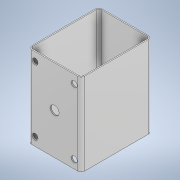
# Autodesk Inventor part: SP21V1 Tubo 40x80x100mm
Saved by Autodesk Inventor 2021.2 (Build 252289000, 289)
## iProperties
Created: 2026-06-02
Part Number: SP21V1 Tubo 40x80x100mm
Material: Aluminum
Document SubType Name: Modeling
Designer: nelso
Density: 2.7 g/cm^3
Appearance: Satin
Author: nelso
Autodesk Inventor part; units mm, degrees
ref_plane "YZ Plane" through (0, 0, 0) normal (1, 0, 0) x (0, 1, 0)
ref_plane "XZ Plane" through (0, 0, 0) normal (0, 1, 0) x (-1, 0, 0)
ref_plane "XY Plane" through (0, 0, 0) normal (0, 0, 1) x (1, 0, 0)
sketch "Sketch1" plane through (0, 0, 0) normal (0, 1, 0) x (-1, 0, 0)
  line L0 (-30, 40) -> (30, 40)
  line L1 (30, 40) -> (30, -40)
  line L2 (30, -40) -> (-30, -40)
  line L3 (-30, -40) -> (-30, 40)
  line L4 (-30, 40) -> (30, -40) construction
  line L5 (30, 40) -> (-30, -40) construction
  line L6 (-28.75, 38.75) -> (28.75, 38.75)
  line L7 (28.75, 38.75) -> (28.75, -38.75)
  line L8 (28.75, -38.75) -> (-28.75, -38.75)
  line L9 (-28.75, -38.75) -> (-28.75, 38.75)
  line L10 (-28.75, 38.75) -> (28.75, -38.75) construction
  line L11 (28.75, 38.75) -> (-28.75, -38.75) construction
  point P0 (0, 0)
  dimension "d0" = 60
  dimension "d1" = 80
  dimension "d2" = 57.5
  dimension "d3" = 77.5
  constraints: 24 end point, 4 midpoint, 4 parallel, 2 horizontal, 2 perpendicular
  measures "d0" distance of L1.end L2.end
  measures "d1" distance of L0.end L1.end
  measures "d2" distance of L7.end L8.end
  measures "d3" distance of L6.end L7.end
extrude "Extrusion1" add sketch "Sketch1" along normal mid plane 93.2
fillet "Fillet1" radius 3.75 4 edges at (30, 0, 40) (-30, 0, 40) (30, 0, -40) (-30, 0, -40)
fillet "Fillet1" radius 2.5 4 edges at (28.75, 0, 38.75) (-28.75, 0, -38.75) (28.75, 0, -38.75) (-28.75, 0, 38.75)
sketch "Sketch3" plane through (26.25, 46.6, -40) normal (0, 0, -1) x (-1, 0, 0)
  circle A0 centre (26.25, -46.6) radius 4.95
  point P0 (26.25, -46.6)
  dimension "d13" = 9.9
  constraints: 1 centre point
  measures "d13" diameter of A0
extrude "Extrusion3" cut sketch "Sketch3" against normal through all
sketch "Sketch15" plane through (-26.25, -46.6, 40) normal (0, 0, 1) x (1, 0, 0)
  arc A0 (44.325, 81.85) -> (52.625, 81.85) centre (48.475, 81.85) ccw projected
  line L0 (44.325, 85.35) -> (44.325, 81.85) projected
  arc A1 (52.625, 85.35) -> (44.325, 85.35) centre (48.475, 85.35) ccw projected
  line L1 (52.625, 81.85) -> (52.625, 85.35) projected
  line L2 (8.175, 81.85) -> (8.175, 85.35) projected
  arc A2 (-0.125, 81.85) -> (8.175, 81.85) centre (4.025, 81.85) ccw projected
  line L3 (-0.125, 85.35) -> (-0.125, 81.85) projected
  arc A3 (8.175, 85.35) -> (-0.125, 85.35) centre (4.025, 85.35) ccw projected
  line L4 (52.625, 7.85) -> (52.625, 11.35) projected
  arc A4 (44.325, 7.85) -> (52.625, 7.85) centre (48.475, 7.85) ccw projected
  line L5 (44.325, 11.35) -> (44.325, 7.85) projected
  arc A5 (52.625, 11.35) -> (44.325, 11.35) centre (48.475, 11.35) ccw projected
  line L6 (-0.125, 11.35) -> (-0.125, 7.85) projected
  arc A6 (8.175, 11.35) -> (-0.125, 11.35) centre (4.025, 11.35) ccw projected
  line L7 (8.175, 7.85) -> (8.175, 11.35) projected
  arc A7 (-0.125, 7.85) -> (8.175, 7.85) centre (4.025, 7.85) ccw projected
  circle A8 centre (26.25, 46.6) radius 18.7446 projected
  arc A9 (56.25, 90.2) -> (53.25, 93.2) centre (53.25, 90.2) ccw projected
  line L8 (-0.75, 93.2) -> (53.25, 93.2) projected
  arc A10 (-0.75, 93.2) -> (-3.75, 90.2) centre (-0.75, 90.2) ccw projected
  line L9 (-3.75, 3) -> (-3.75, 90.2) projected
  arc A11 (-3.75, 3) -> (-0.75, 0) centre (-0.75, 3) ccw projected
  line L10 (53.25, 0) -> (-0.75, 0) projected
  arc A12 (53.25, 0) -> (56.25, 3) centre (53.25, 3) ccw projected
  line L11 (56.25, 90.2) -> (56.25, 3) projected
  line L12 (4.025, 81.85) -> (4.025, 85.35)
  line L13 (48.475, 81.85) -> (48.475, 85.35)
  line L14 (48.475, 7.85) -> (48.475, 11.35)
  line L15 (4.025, 7.85) -> (4.025, 11.35)
  point P0 (26.25, 46.6)
  point P1 (4.025, 9.6)
  point P2 (48.475, 9.6)
  point P3 (48.475, 83.6)
  point P4 (4.025, 83.6)
  constraints: 8 end point, 4 midpoint, 4 vertical
hole "Hole1" at (-22.225, -37, 40) at (22.225, -37, 40) at (22.225, 37, 40) at (-22.225, 37, 40) direction (0, 0, -1) diameter 6.6 depth 8 tip angle 118 clearance for "Countersunk Flat Head Screw ISO 2009/7046" size "M6" standard "ISO"
sketch "Sketch16" plane through (26.25, 46.6, -40) normal (0, 0, -1) x (-1, 0, 0)
  line L0 (0, 0) -> (0, -93.2) projected
  line L1 (52.5, 0) -> (52.5, -93.2) projected
  line L2 (0, -93.2) -> (52.5, -93.2)
  line L3 (52.5, -93.2) -> (52.5, -63.2)
  line L4 (52.5, -63.2) -> (0, -63.2)
  line L5 (0, -63.2) -> (0, -93.2)
  point P0 (26.25, -46.6)
  point P1 (0, -63.2)
  dimension "d59" = 30
  constraints: 8 end point, 2 parallel, 1 horizontal, 1 perpendicular, 1 point on line
  measures "d59" distance of L3.end L2.end
extrude "Extrusion15" cut sketch "Sketch16" against normal blind 10
fillet "Fillet3" radius 2 4 edges at (26.25, -46.6, -39.375) (26.25, -16.6, -39.375) (-26.25, -46.6, -39.375) (-26.25, -16.6, -39.375)
body "Solid1"
